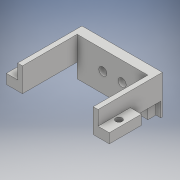
# Autodesk Inventor part: soporteCamaraA
Saved by Autodesk Inventor 2017 (Build 210142000, 142)
## iProperties
Part Number: soporteCamaraA
Material: Genérico
Document SubType Name: Modeling
Designer: Roberto
Density: 1 g/cm^3
Appearance: Valor por defecto
Author: Roberto
Autodesk Inventor part; units mm, degrees
ref_plane "YZ Plane" through (0, 0, 0) normal (1, 0, 0) x (0, 1, 0)
sketch "Boceto1" plane through (0, 0, 0) normal (0, 1, 0) x (-1, 0, 0)
  line L0 (0, 0) -> (1.35, 0)
  line L1 (1.35, 0) -> (1.35, -1.2)
  line L2 (1.35, -1.2) -> (-1.35, -1.2)
  line L3 (-1.35, -1.2) -> (-1.35, 0)
  line L4 (-1.35, 0) -> (0, 0)
  circle A0 centre (0.3, -0.6) radius 0.125
  circle A1 centre (-0.3, -0.6) radius 0.125
  dimension "d4" = 1.35
  dimension "d5" = 1.2
  dimension "d6" = 2.7
  dimension "d7" = 1.2
  constraints: 10 end point, 2 centre point, 2 perpendicular, 1 horizontal, 1 vertical
  measures "d4" distance of L0.start L0.end
  measures "d5" distance of L0.end L1.end
  measures "d6" distance of L1.end L2.end
  measures "d7" distance of L2.end L3.end
extrude "Extrusión1" add sketch "Boceto1" against normal blind 0.3
sketch "Boceto6" plane through (0, -0.3, 0) normal (0, -1, 0) x (1, 0, 0)
  line L0 (1.35, 0) -> (-1.35, 0) projected
  line L1 (-1.35, 0) -> (-1.35, -1.2) projected
  line L2 (-1.35, -1.2) -> (1.35, -1.2) projected
  line L3 (1.35, -1.2) -> (1.35, 0) projected
  line L4 (1.1, -1.2) -> (1.1, 0)
  line L5 (-1.1, -1.2) -> (-1.1, 0)
  line L6 (1.35, 0) -> (-1.35, 0) projected
  line L7 (1.25, 0) -> (1.1, 0)
  line L8 (1.1, 0) -> (1.1, -1.2)
  line L9 (1.1, -1.2) -> (1.25, -1.2)
  line L10 (1.25, -1.2) -> (1.25, 0)
  line L11 (-1.1, -1.2) -> (-1.25, -1.2)
  line L12 (-1.25, -1.2) -> (-1.25, 0)
  line L13 (-1.25, 0) -> (-1.1, 0)
  line L14 (-1.1, 0) -> (-1.1, -1.2)
  line L15 (-1.35, -1.2) -> (1.35, -1.2) projected
  line L16 (-1.25, -1.2) -> (-1.35, -1.2)
  line L17 (-1.35, -1.2) -> (-1.35, 0)
  line L18 (-1.35, 0) -> (-1.25, 0)
  line L19 (-1.25, 0) -> (-1.25, -1.2)
  line L20 (1.35, -1.2) -> (1.25, -1.2)
  line L21 (1.25, -1.2) -> (1.25, 0)
  line L22 (1.25, 0) -> (1.35, 0)
  line L23 (1.35, 0) -> (1.35, -1.2)
  point P0 (0, 0)
  constraints: 36 end point, 9 parallel, 5 perpendicular, 4 horizontal, 2 point on line
extrude "Extrusión5" add sketch "Boceto6" along normal blind 1.7 contours L3 L2 L10 L0 | L10 L2 L4 L0 | L5 L2 L12 L0 | L12 L2 L1 L0
ref_plane "Plano de trabajo3" through (1.35, 0, -2.8) normal (0, 0, -1) x (-1, 0, 0)
sketch "Boceto9" plane through (1.35, 0, -1.2) normal (0, 0, -1) x (-1, 0, 0)
  line L0 (0.1, -2.25) -> (0.1, -1.25) projected
  line L1 (2.6, -1.25) -> (2.6, -2.25) projected
  line L2 (2.7, 0) -> (2.7, -2) projected
  line L3 (0, 0) -> (0, -2) projected
  line L4 (0.1, -2.25) -> (0, -2.25)
  line L5 (0, -2.25) -> (0, 0)
  line L6 (0, 0) -> (0.1, 0)
  line L7 (0.1, 0) -> (0.1, -2.25)
  line L8 (2.6, -2.25) -> (2.7, -2.25)
  line L9 (2.7, -2.25) -> (2.7, 0)
  line L10 (2.7, 0) -> (2.6, 0)
  line L11 (2.6, 0) -> (2.6, -2.25)
  point P0 (1.35, 0)
  constraints: 16 end point, 4 parallel, 2 horizontal, 2 perpendicular
extrude "Extrusión8" cut sketch "Boceto9" against normal blind 4
ref_plane "Plano de trabajo1" through (0, 0, -0.6) normal (0, 0, 1) x (1, 0, 0)
sketch "Boceto11" plane through (0, 0, -0.6) normal (0, 0, 1) x (1, 0, 0)
  circle A0 centre (1.4, -1.75) radius 0.1 projected
  line L0 (1.6, -1.25) -> (1.25, -1.25) projected
  line L1 (1.25, -2.25) -> (1.6, -2.25) projected
  line L2 (1.6, -2.25) -> (1.6, -1.25) projected
  line L3 (-1.1, -1.25) -> (-1.6, -1.25) projected
  line L4 (-1.6, -1.25) -> (-1.6, -2.25) projected
  line L5 (-1.6, -2.25) -> (-1.1, -2.25) projected
  circle A1 centre (-1.4, -1.75) radius 0.1 projected
  line L6 (-1.1, -2.25) -> (-1.1, -1.25) projected
  line L7 (1.25, -1.25) -> (1.25, -2.25) projected
  line L8 (1.1, -2) -> (1.25, -2) projected
  line L9 (1.25, -1.25) -> (1.6, -1.25)
  line L10 (-1.6, -1.25) -> (-1.1, -1.25)
  circle A2 centre (1.4, -1.75) radius 0.1
  line L11 (1.25, -1) -> (1.6, -1)
  line L12 (1.6, -1) -> (1.6, -2)
  line L13 (1.6, -2) -> (1.25, -2)
  line L14 (1.25, -2) -> (1.25, -1)
  line L15 (-1.6, -1) -> (-1.1, -1)
  line L16 (-1.1, -1) -> (-1.1, -2)
  line L17 (-1.1, -2) -> (-1.6, -2)
  line L18 (-1.6, -2) -> (-1.6, -1)
  circle A3 centre (-1.4, -1.5) radius 0.1
  circle A4 centre (1.4, -1.5) radius 0.1
  point P0 (0, 0)
  constraints: 20 end point, 4 horizontal, 4 parallel, 3 centre point, 2 perpendicular, 1 coincident, 1 concentric
extrude "Extrusión9" add sketch "Boceto11" along normal mid plane 0.3 contours A0 | L2 L13 L7 L0 | L0 L14 L11 L12 | L6 L17 L4 L3 | L3 L18 L15 L16 | A1
sketch "Boceto12" plane through (0, -2, 0) normal (0, -1, 0) x (1, 0, 0)
  line L0 (-1.25, -0.75) -> (-1.25, -1.2) projected
  line L1 (1.25, -1.2) -> (1.25, -0.75) projected
  line L2 (1.1, -1.2) -> (1.25, -1.2) projected
  line L3 (-1.25, -1.2) -> (-1.1, -1.2) projected
  line L4 (-1.25, -0.75) -> (-1.1, -0.75)
  line L5 (-1.1, -0.75) -> (-1.1, -1.2)
  line L6 (-1.1, -1.2) -> (-1.25, -1.2)
  line L7 (-1.25, -1.2) -> (-1.25, -0.75)
  line L8 (1.25, -0.75) -> (1.1, -0.75)
  line L9 (1.1, -0.75) -> (1.1, -1.2)
  line L10 (1.1, -1.2) -> (1.25, -1.2)
  line L11 (1.25, -1.2) -> (1.25, -0.75)
  point P0 (0, 0)
  constraints: 16 end point, 4 parallel, 2 horizontal, 2 perpendicular
extrude "Extrusión10" cut sketch "Boceto12" against normal blind 1.95
